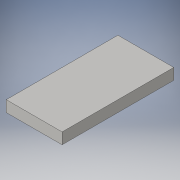
# Autodesk Inventor part: bottomOfCase
Saved by Autodesk Inventor 2016 (Build 200138000, 138)
## iProperties
Created: 2015-09-19
Part Number: bottomOfCase
Material: Generic
Document SubType Name: Modeling
Designer: steele
Density: 1 g/cm^3
Appearance: Default
Author: steele
Autodesk Inventor part; units mm, degrees
ref_plane "YZ Plane" through (0, 0, 0) normal (1, 0, 0) x (0, 1, 0)
ref_plane "XZ Plane" through (0, 0, 0) normal (0, 1, 0) x (-1, 0, 0)
ref_plane "XY Plane" through (0, 0, 0) normal (0, 0, 1) x (1, 0, 0)
sketch "Sketch1" plane through (0, 0, 0) normal (0, 1, 0) x (-1, 0, 0)
  line L0 (-63.5, 127) -> (-63.5, -127)
  line L1 (-63.5, -127) -> (63.5, -127)
  line L2 (63.5, -127) -> (63.5, 127)
  line L3 (63.5, 127) -> (-63.5, 127)
  line L4 (-63.5, 127) -> (63.5, -127) construction
  line L5 (-63.5, -127) -> (63.5, 127) construction
  point P0 (0, 0)
  dimension "height" = 127
  dimension "width" = 254
  constraints: 12 end point, 2 midpoint, 2 parallel, 1 perpendicular, 1 vertical
  measures "height" distance of L2.end L0.start
  measures "width" distance of L1.end L2.end
extrude "Extrusion1" add sketch "Sketch1" along normal blind 25.4
body "Solid1"
